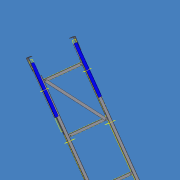
# Autodesk Inventor part: Part1
Saved by Autodesk Inventor 2015 (Build 190159000, 159)
## iProperties
Created: 2007-08-01
Part Number: Part1
Material: Steel, Mild
Document SubType Name: Modeling
Designer: kurt
Manufacturer: Standard
Standards Organization: Custom
Density: 7.86 g/cm^3
Appearance: Steel
Behandeling: Behandeling
Besteld: S
Materiaal: st37
Totaal: 0
Author: kurt
Autodesk Inventor part; units mm, degrees
ref_plane "YZ Plane" through (0, 0, 0) normal (1, 0, 0) x (0, 1, 0)
ref_plane "XZ Plane" through (0, 0, 0) normal (0, 1, 0) x (-1, 0, 0)
ref_plane "XY Plane" through (0, 0, 0) normal (0, 0, 1) x (1, 0, 0)
sketch "Sketch1" plane through (0, 0, 0) normal (0, 0, 1) x (1, 0, 0)
  circle A0 centre (190.0545, 3.9636) radius 5.5 projected
  circle A1 centre (-96.9878, 447.3295) radius 5.5 projected
  arc A2 (177.463, -4.1883) -> (202.646, 12.1156) centre (190.0545, 3.9636) ccw
  arc A3 (-84.3963, 455.4815) -> (-109.5793, 439.1776) centre (-96.9878, 447.3295) ccw
  line L0 (-84.3963, 455.4815) -> (202.646, 12.1156)
  line L1 (177.463, -4.1883) -> (-109.5793, 439.1776)
  circle A4 centre (190.0545, 3.9636) radius 5.5
  circle A5 centre (-96.9878, 447.3295) radius 5.5
  point P0 (0, 0)
  dimension "d2" = 30
  dimension "d3" = 30
  dimension "d4" = 11
  dimension "d5" = 11
  constraints: 4 centre point, 4 coincident, 4 end point, 4 point on circle, 4 tangent
  measures "d2" diameter of A2
  measures "d3" diameter of A3
  measures "d4" diameter of A4
  measures "d5" diameter of A5
extrude "Extrusion2" add sketch "Sketch1" along normal blind 6
body "Solid1"
